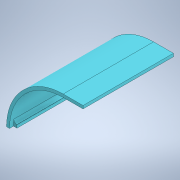
# Autodesk Inventor part: obudowa przekładni 2
Saved by Autodesk Inventor 2021 (Build 250183000, 183)
## iProperties
Created: 2022-01-26
Part Number: obudowa przekładni 2
Material: Generic
Document SubType Name: Modeling
Designer: Łukasz
Density: 1 g/cm^3
Appearance: Cadet Blue
Author: Łukasz
Autodesk Inventor part; units mm, degrees
ref_plane "YZ Plane" through (0, 0, 0) normal (1, 0, 0) x (0, 1, 0)
ref_plane "XZ Plane" through (0, 0, 0) normal (0, 1, 0) x (-1, 0, 0)
ref_plane "XY Plane" through (0, 0, 0) normal (0, 0, 1) x (1, 0, 0)
sketch "Sketch1" plane through (0, 0, 0) normal (0, 0, 1) x (1, 0, 0)
  arc A0 (0, 54) -> (-54, 0) centre (0, 0) ccw
  arc A1 (0, 57) -> (-57, 0) centre (0, 0) ccw
  line L0 (0, 57) -> (20, 57)
  line L1 (0, 57) -> (20, 57) construction
  line L2 (0, 54) -> (20, 54)
  line L3 (0, 54) -> (20, 54) construction
  line L4 (20, 54) -> (20, 57)
  line L5 (-57, 0) -> (-54, 0)
  dimension "d0" = 108
  dimension "d1" = 114
  dimension "d2" = 20
  dimension "d3" = 0
  dimension "d4" = 20
  dimension "d5" = 0
  constraints: 12 end point, 5 horizontal, 4 point on circle, 2 centre point, 2 coincident, 2 collinear, 2 tangent
  measures "d0" diameter of A0
  measures "d1" diameter of A1
  measures "d2" distance of L0.start L0.end
  measures "d3" distance between parallel lines of L0 L1
  measures "d4" distance of L2.start L2.end
  measures "d5" distance between parallel lines of L2 L3
extrude "Extrusion1" add sketch "Sketch1" along normal blind 91
sketch "Sketch2" plane through (-57, 0, 0) normal (0, -1, 0) x (1, 0, 0)
  line L0 (3, 0) -> (3, 91) projected
  line L1 (3, 87) -> (6.5, 87)
  line L2 (6.5, 87) -> (6.5, 4)
  line L3 (6.5, 4) -> (3, 4)
  line L4 (3, 4) -> (3, 87)
  line L5 (0, 0) -> (3, 0) projected
  point P0 (57, 0)
  point P1 (3, 4)
  dimension "d8" = 3.5
  dimension "d9" = 83
  dimension "d10" = 4
  constraints: 8 end point, 2 parallel, 1 horizontal, 1 perpendicular, 1 point on line
  measures "d8" distance of L2.end L3.end
  measures "d9" distance of L1.end L2.end
  measures "d10" distance between parallel lines of L5 L3
extrude "Extrusion2" add sketch "Sketch2" against normal blind 3
fillet "Fillet1" radius 3 1 edges at (-53.9166, 3, 45.5)
body "Solid1"
